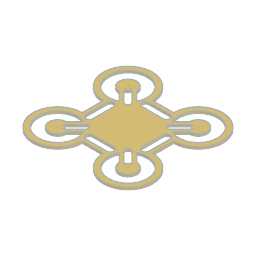
drone (Autodesk Fusion 360 archive; units mm, degrees)
design "body"
part number: 2026-07-30-17-30-24-029
Autodesk Fusion 360 part; units mm, degrees
sketch "Sketch1" plane through (0, 0, 0) normal (0, 1, 0) x (1, 0, 0)
  circle A0 centre (0, 0) radius 35
  circle A1 centre (100, 0.0136) radius 35
  circle A2 centre (0, 100) radius 35
  circle A3 centre (100.1584, 100.0135) radius 35
  line L0 (0, 0) -> (100.1584, 0)
  line L1 (100.1584, 0) -> (100.1584, 100.0135)
  line L2 (100.1584, 100.0135) -> (0, 100.0135)
  line L3 (0, 100.0135) -> (0, 0)
  circle A4 centre (0, 0) radius 27.5
  circle A5 centre (100, 0.0136) radius 27.5
  circle A6 centre (100.1584, 100.0135) radius 27.5
  circle A7 centre (0, 100) radius 27.5
  circle A8 centre (100.1584, 100.0135) radius 12.5
  circle A9 centre (0, 100) radius 12.5
  circle A10 centre (100, 0.0136) radius 12.5
  circle A11 centre (0, 0) radius 12.5
  line L4 (0, 12.5) -> (21.9203, 34.4203)
  line L5 (21.9203, 34.4203) -> (34.4203, 21.9203)
  line L6 (34.4203, 21.9203) -> (12.5, 0)
  line L7 (0, 12.5) -> (12.5, 0)
  line L8 (87.5, 0) -> (65.707, 22.0469)
  line L9 (65.707, 22.0469) -> (78.3654, 34.5595)
  line L10 (78.3654, 34.5595) -> (100.1584, 12.5126)
  line L11 (87.5, 0) -> (100.1584, 12.5126)
  line L12 (0, 87.5) -> (12.5, 100.0135)
  line L13 (0, 87.5) -> (21.9321, 65.5915)
  line L14 (21.9321, 65.5915) -> (34.4321, 78.105)
  line L15 (34.4321, 78.105) -> (12.5, 100.0135)
  line L16 (87.6584, 100.0135) -> (100.1584, 87.5135)
  line L17 (100.1584, 87.5135) -> (78.2381, 65.5932)
  line L18 (87.6584, 100.0135) -> (65.7381, 78.0932)
  line L19 (65.7381, 78.0932) -> (78.2381, 65.5932)
  dimension "d1" = 70
  dimension "d2" = 70
  dimension "d3" = 70
  dimension "d4" = 70
  dimension "d5" = 100
  dimension "d6" = 100
  dimension "d7" = 100
  dimension "d8" = 55
  dimension "d9" = 55
  dimension "d10" = 55
  dimension "d11" = 55
  dimension "d12" = 25
  dimension "d13" = 25
  dimension "d14" = 25
  dimension "d15" = 25
  dimension "d16" = 31
  dimension "d17" = 31
  dimension "d18" = 31
  dimension "d19" = 31
  constraint coincident A0.centre L0.start
  constraint horizontal L0
  constraint vertical L1
  constraint horizontal L2
  constraint vertical L3
  constraint coincident A3.centre L1.end
  constraint concentric A0 A4
  constraint concentric A1 A5
  constraint concentric A3 A6
  constraint concentric A2 A7
  constraint concentric A3 A8
  constraint concentric A2 A9
  constraint concentric A5 A10
  constraint coincident L3 L4.start
  constraint coincident A11 L4.start
  constraint coincident A11 L6.end
  constraint coincident L0 L6.end
  constraint perpendicular L5 L6
  constraint perpendicular L4 L5
  constraint parallel L5 L7
  constraint coincident A10 L8.start
  constraint coincident L0 L8.start
  constraint coincident A10 L10.end
  constraint coincident L1 L10.end
  constraint parallel L9 L11
  constraint perpendicular L8 L11
  constraint perpendicular L9 L10
  constraint coincident A9 L12.start
  constraint coincident L3 L12.start
  constraint coincident A9 L12.end
  constraint coincident L2 L12.end
  constraint perpendicular L12 L13
  constraint perpendicular L13 L14
  constraint perpendicular L14 L15
  constraint coincident A8 L16.start
  constraint coincident L2 L16.start
  constraint coincident L1 L16.end
  constraint coincident A8 L16.end
  constraint coincident L16 L18.start
  constraint perpendicular L18 L19
  constraint perpendicular L17 L19
  constraint parallel L16 L19
  measures "d1" diameter of A0
  measures "d2" diameter of A1
  measures "d3" diameter of A2
  measures "d4" diameter of A3
  measures "d5" distance of A1.centre A3.centre
  measures "d6" distance of A0.centre A1.centre
  measures "d7" distance of A0.centre A2.centre
  measures "d8" diameter of A4
  measures "d9" diameter of A5
  measures "d10" diameter of A6
  measures "d11" diameter of A7
  measures "d12" diameter of A8
  measures "d13" diameter of A9
  measures "d14" diameter of A10
  measures "d15" diameter of A11
  measures "d16" distance of L5.end L6.end
  measures "d17" distance of L8.start L8.end
  measures "d18" distance of L12.end L14.end
  measures "d19" distance of L16.end L17.end
extrude "Extrude1" add sketch "Sketch1" along normal blind 3 contours A0 L0 A4 L6 | A0 L0 L3 A4 | A0 A1 A2 A3 L0 L1 L2 L3 L4 L5 L6 L8 L9 L10 L13 L14 L15 L17 L18 L19 | A0 A4 L4 L6 | A0 L4 L5 L6 | A0 L3 A4 L4 | A1 L0 L1 A5 | A1 L0 A5 L8 | A4 A11 L4 L6 | A2 L3 A7 L13 | A2 L2 L3 A7 | L0 L3 A11 | A11 L7 | L0 L3 L7 | A1 L8 L9 L10 | A1 A5 L8 L10 | A2 L2 A7 L15 | A2 A7 L13 L15 | A2 L13 L14 L15 | A1 L1 A5 L10 | A5 A10 L8 L10 | L0 L1 L11 | L0 L1 A10 | A10 L11 | A3 L2 A6 L18 | A3 L1 L2 A6 | A7 A9 L13 L15 | L2 L3 A9 | A9 L12 | L2 L3 L12 | A3 L1 A6 L17 | A3 A6 L17 L18 | A3 L17 L18 L19 | A6 A8 L17 L18 | L1 L2 A8 | A8 L16 | L1 L2 L16
move_face "MoveFace1" by (0, 0, 90) 1 faces at (58.5153, 0, -62.6556)
move_body "Move1" bodies 1 to x (1, 0, 0) y (0, 0, -1) z (0, 1, 0) at (0, 49.9918, 80.0082)
sketch "Sketch2" plane through (0, 0, 80.0082) normal (0, 0, 1) x (-1, 0, 0)
  line L0 (-100.1584, 37.5217) -> (-87.9948, 25.3581)
  arc A0 (-75.4948, 37.8581) -> (-87.9948, 25.3581) centre (-100.1584, 50.0217) ccw
  line L1 (-75.4948, 37.8581) -> (-87.6584, 50.0217)
  arc A1 (-87.6584, 50.0217) -> (-100.1584, 37.5217) centre (-100.1584, 50.0217) ccw
  line L2 (0, -37.4918) -> (-12.1636, -25.3281)
  arc A2 (-24.6636, -37.8281) -> (-12.1636, -25.3281) centre (0, -49.9918) ccw
  line L3 (-24.6636, -37.8281) -> (-12.5, -49.9918)
  arc A3 (-12.5, -49.9918) -> (0, -37.4918) centre (0, -49.9918) ccw
  line L4 (-12.5, 50.0217) -> (-24.6724, 37.8624)
  arc A4 (-12.1725, 25.3489) -> (-24.6724, 37.8624) centre (0, 50.0082) ccw
  line L5 (-12.1725, 25.3489) -> (0, 37.5082)
  arc A5 (0, 37.5082) -> (-12.5, 50.0217) centre (0, 50.0082) ccw
  line L6 (-87.5, -49.9918) -> (-75.3786, -37.7292)
  arc A6 (-88.037, -25.2165) -> (-75.3786, -37.7292) centre (-100, -49.9781) ccw
  line L7 (-88.037, -25.2165) -> (-100.1584, -37.4791)
  arc A7 (-100.1584, -37.4791) -> (-87.5, -49.9918) centre (-100, -49.9781) ccw
  arc A8 (0, 15.0082) -> (-35, 50.0217) centre (0, 50.0082) ccw
  line L8 (-35, 50.0217) -> (-65.1584, 50.0217)
  arc A9 (-65.1584, 50.0217) -> (-100.1584, 15.0217) centre (-100.1584, 50.0217) ccw
  line L9 (-100.1584, 15.0217) -> (-100.1584, -14.9785)
  arc A10 (-100.1584, -14.9785) -> (-65, -49.9918) centre (-100, -49.9781) ccw
  line L10 (-65, -49.9918) -> (-35, -49.9918)
  arc A11 (-35, -49.9918) -> (0, -14.9918) centre (0, -49.9918) ccw
  line L11 (0, -14.9918) -> (0, 15.0082)
  line L12 (-35, -35) -> (-65, -35)
  arc A12 (-65, -35) -> (-65, -45) centre (-65, -40) ccw
  line L13 (-65, -45) -> (-35, -45)
  arc A13 (-35, -45) -> (-35, -35) centre (-35, -40) ccw
  line L14 (-35, -40) -> (-65, -40) construction
  line L15 (-35, 45) -> (-65, 45)
  arc A14 (-65, 45) -> (-65, 35) centre (-65, 40) ccw
  line L16 (-65, 35) -> (-35, 35)
  arc A15 (-35, 35) -> (-35, 45) centre (-35, 40) ccw
  line L17 (-35, 40) -> (-65, 40) construction
  line L18 (-15, 15) -> (-15, -15)
  arc A16 (-15, -15) -> (-5, -15) centre (-10, -15) ccw
  line L19 (-5, -15) -> (-5, 15)
  arc A17 (-5, 15) -> (-15, 15) centre (-10, 15) ccw
  line L20 (-10, 15) -> (-10, -15) construction
  line L21 (-95, 15) -> (-95, -15)
  arc A18 (-95, -15) -> (-85, -15) centre (-90, -15) ccw
  line L22 (-85, -15) -> (-85, 15)
  arc A19 (-85, 15) -> (-95, 15) centre (-90, 15) ccw
  line L23 (-90, 15) -> (-90, -15) construction
  dimension "d22" = 10
  dimension "d23" = 10
  constraint tangent L12 A12
  constraint tangent A12 L13
  constraint parallel L12 L13
  constraint tangent L13 A13
  constraint tangent L12 A13
  constraint horizontal L14
  constraint tangent L15 A14
  constraint tangent A14 L16
  constraint parallel L15 L16
  constraint tangent L16 A15
  constraint tangent L15 A15
  constraint parallel L12 L17
  constraint tangent L18 A16
  constraint tangent A16 L19
  constraint parallel L18 L19
  constraint tangent L19 A17
  constraint tangent L18 A17
  constraint vertical L20
  constraint tangent L21 A18
  constraint tangent A18 L22
  constraint parallel L21 L22
  constraint tangent L22 A19
  constraint tangent L21 A19
  constraint parallel L9 L23
  measures "d22" diameter of A14
  measures "d23" diameter of A18
extrude "Extrude2" cut sketch "Sketch2" against normal blind 40 contours L12 A12 L13 A13 | L15 A14 L16 A15 | L18 A16 L19 A17 | L21 A18 L22 A19
sketch "Sketch3" plane through (0, 0, 80.0082) normal (0, 0, 1) x (-1, 0, 0)
  arc A0 (0, 15.0082) -> (-35, 50.0217) centre (0, 50.0082) ccw
  line L0 (-35, 50.0217) -> (-65.1584, 50.0217)
  arc A1 (-65.1584, 50.0217) -> (-100.1584, 15.0217) centre (-100.1584, 50.0217) ccw
  line L1 (-100.1584, 15.0217) -> (-100.1584, -14.9785)
  arc A2 (-100.1584, -14.9785) -> (-65, -49.9918) centre (-100, -49.9781) ccw
  line L2 (-65, -49.9918) -> (-35, -49.9918)
  arc A3 (-35, -49.9918) -> (0, -14.9918) centre (0, -49.9918) ccw
  line L3 (0, -14.9918) -> (0, 15.0082)
  line L4 (-87.5, -49.9918) -> (-75.3786, -37.7292)
  arc A4 (-88.037, -25.2165) -> (-75.3786, -37.7292) centre (-100, -49.9781) ccw
  line L5 (-88.037, -25.2165) -> (-100.1584, -37.4791)
  arc A5 (-100.1584, -37.4791) -> (-87.5, -49.9918) centre (-100, -49.9781) ccw
  line L6 (-12.5, 50.0217) -> (-24.6724, 37.8624)
  arc A6 (-12.1725, 25.3489) -> (-24.6724, 37.8624) centre (0, 50.0082) ccw
  line L7 (-12.1725, 25.3489) -> (0, 37.5082)
  arc A7 (0, 37.5082) -> (-12.5, 50.0217) centre (0, 50.0082) ccw
  line L8 (0, -37.4918) -> (-12.1636, -25.3281)
  arc A8 (-24.6636, -37.8281) -> (-12.1636, -25.3281) centre (0, -49.9918) ccw
  line L9 (-24.6636, -37.8281) -> (-12.5, -49.9918)
  arc A9 (-12.5, -49.9918) -> (0, -37.4918) centre (0, -49.9918) ccw
  line L10 (-100.1584, 37.5217) -> (-87.9948, 25.3581)
  arc A10 (-75.4948, 37.8581) -> (-87.9948, 25.3581) centre (-100.1584, 50.0217) ccw
  line L11 (-75.4948, 37.8581) -> (-87.6584, 50.0217)
  arc A11 (-87.6584, 50.0217) -> (-100.1584, 37.5217) centre (-100.1584, 50.0217) ccw
  line L12 (-65, 45) -> (-35, 45)
  arc A12 (-35, 35) -> (-35, 45) centre (-35, 40) ccw
  line L13 (-35, 35) -> (-65, 35)
  arc A13 (-65, 45) -> (-65, 35) centre (-65, 40) ccw
  line L14 (-95, -15) -> (-95, 15)
  arc A14 (-85, 15) -> (-95, 15) centre (-90, 15) ccw
  line L15 (-85, 15) -> (-85, -15)
  arc A15 (-95, -15) -> (-85, -15) centre (-90, -15) ccw
  line L16 (-15, -15) -> (-15, 15)
  arc A16 (-5, 15) -> (-15, 15) centre (-10, 15) ccw
  line L17 (-5, 15) -> (-5, -15)
  arc A17 (-15, -15) -> (-5, -15) centre (-10, -15) ccw
  line L18 (-65, -35) -> (-35, -35)
  arc A18 (-35, -45) -> (-35, -35) centre (-35, -40) ccw
  line L19 (-35, -45) -> (-65, -45)
  arc A19 (-65, -35) -> (-65, -45) centre (-65, -40) ccw
  line L20 (-7.8284, 47.8284) -> (-22.8284, 32.8284)
  arc A20 (-22.8284, 32.8284) -> (-17.1716, 27.1716) centre (-20, 30) ccw
  line L21 (-17.1716, 27.1716) -> (-2.1716, 42.1716)
  arc A21 (-2.1716, 42.1716) -> (-7.8284, 47.8284) centre (-5, 45) ccw
  line L22 (-5, 45) -> (-20, 30) construction
  line L23 (-97.8284, 42.1716) -> (-82.8284, 27.1716)
  arc A22 (-82.8284, 27.1716) -> (-77.1716, 32.8284) centre (-80, 30) ccw
  line L24 (-77.1716, 32.8284) -> (-92.1716, 47.8284)
  arc A23 (-92.1716, 47.8284) -> (-97.8284, 42.1716) centre (-95, 45) ccw
  line L25 (-95, 45) -> (-80, 30) construction
  line L26 (-92.1552, -47.812) -> (-77.2438, -32.7268)
  arc A24 (-77.2438, -32.7268) -> (-82.9333, -27.1028) centre (-80.0885, -29.9148) ccw
  line L27 (-82.9333, -27.1028) -> (-97.8448, -42.188)
  arc A25 (-97.8448, -42.188) -> (-92.1552, -47.812) centre (-95, -45) ccw
  line L28 (-95, -45) -> (-80.0885, -29.9148) construction
  line L29 (-2.1716, -42.1716) -> (-17.1716, -27.1716)
  arc A26 (-17.1716, -27.1716) -> (-22.8284, -32.8284) centre (-20, -30) ccw
  line L30 (-22.8284, -32.8284) -> (-7.8284, -47.8284)
  arc A27 (-7.8284, -47.8284) -> (-2.1716, -42.1716) centre (-5, -45) ccw
  line L31 (-5, -45) -> (-20, -30) construction
  line L32 (-5, -45) -> (-2.1716, -42.1716)
  line L33 (-5, -45) -> (-7.8284, -47.8284)
  line L34 (-95, -45) -> (-92.1552, -47.812)
  line L35 (-95, -45) -> (-97.8448, -42.188)
  line L36 (-95, 45) -> (-92.1716, 47.8284)
  line L37 (-95, 45) -> (-97.8284, 42.1716)
  line L38 (-5, 45) -> (-7.8284, 47.8284)
  line L39 (-5, 45) -> (-2.1716, 42.1716)
  dimension "d26" = 8
  dimension "d27" = 8
  dimension "d28" = 8
  dimension "d29" = 8
  constraint tangent L20 A20
  constraint tangent A20 L21
  constraint parallel L20 L21
  constraint tangent L21 A21
  constraint tangent L20 A21
  constraint tangent L23 A22
  constraint tangent A22 L24
  constraint parallel L23 L24
  constraint tangent L24 A23
  constraint tangent L23 A23
  constraint tangent L26 A24
  constraint tangent A24 L27
  constraint parallel L26 L27
  constraint tangent L27 A25
  constraint tangent L26 A25
  constraint parallel L4 L28
  constraint tangent L29 A26
  constraint tangent A26 L30
  constraint parallel L29 L30
  constraint tangent L30 A27
  constraint tangent L29 A27
  constraint coincident A27.centre L31.start
  constraint coincident A25.centre L28.start
  constraint coincident A23.centre L25.start
  constraint coincident A21.centre L22.start
  measures "d26" diameter of A20
  measures "d27" diameter of A22
  measures "d28" diameter of A24
  measures "d29" diameter of A26
extrude "Extrude3" cut sketch "Sketch3" against normal blind 3 contours L20 A20 L21 L38 L39 | L23 A22 L24 L36 L37 | L26 A24 L27 L34 L35 | L29 A26 L30 L32 L33
sketch "Sketch4" plane through (0, 0, 80.0082) normal (0, 0, 1) x (-1, 0, 0)
  line L0 (-65, -35) -> (-35, -35)
  arc A0 (-35, -45) -> (-35, -35) centre (-35, -40) ccw
  line L1 (-35, -45) -> (-65, -45)
  arc A1 (-65, -35) -> (-65, -45) centre (-65, -40) ccw
  line L2 (-15, -15) -> (-15, 15)
  arc A2 (-5, 15) -> (-15, 15) centre (-10, 15) ccw
  line L3 (-5, 15) -> (-5, -15)
  arc A3 (-15, -15) -> (-5, -15) centre (-10, -15) ccw
  line L4 (-95, -15) -> (-95, 15)
  arc A4 (-85, 15) -> (-95, 15) centre (-90, 15) ccw
  line L5 (-85, 15) -> (-85, -15)
  arc A5 (-95, -15) -> (-85, -15) centre (-90, -15) ccw
  line L6 (-65, 45) -> (-35, 45)
  arc A6 (-35, 35) -> (-35, 45) centre (-35, 40) ccw
  line L7 (-35, 35) -> (-65, 35)
  arc A7 (-65, 45) -> (-65, 35) centre (-65, 40) ccw
  line L8 (-100.1584, 37.5217) -> (-87.9948, 25.3581)
  arc A8 (-75.4948, 37.8581) -> (-87.9948, 25.3581) centre (-100.1584, 50.0217) ccw
  line L9 (-75.4948, 37.8581) -> (-87.6584, 50.0217)
  arc A9 (-87.6584, 50.0217) -> (-100.1584, 37.5217) centre (-100.1584, 50.0217) ccw
  line L10 (0, -37.4918) -> (-12.1636, -25.3281)
  arc A10 (-24.6636, -37.8281) -> (-12.1636, -25.3281) centre (0, -49.9918) ccw
  line L11 (-24.6636, -37.8281) -> (-12.5, -49.9918)
  arc A11 (-12.5, -49.9918) -> (0, -37.4918) centre (0, -49.9918) ccw
  line L12 (-12.5, 50.0217) -> (-24.6724, 37.8624)
  arc A12 (-12.1725, 25.3489) -> (-24.6724, 37.8624) centre (0, 50.0082) ccw
  line L13 (-12.1725, 25.3489) -> (0, 37.5082)
  arc A13 (0, 37.5082) -> (-12.5, 50.0217) centre (0, 50.0082) ccw
  line L14 (-87.5, -49.9918) -> (-75.3786, -37.7292)
  arc A14 (-88.037, -25.2165) -> (-75.3786, -37.7292) centre (-100, -49.9781) ccw
  line L15 (-88.037, -25.2165) -> (-100.1584, -37.4791)
  arc A15 (-100.1584, -37.4791) -> (-87.5, -49.9918) centre (-100, -49.9781) ccw
  arc A16 (0, 15.0082) -> (-35, 50.0217) centre (0, 50.0082) ccw
  line L16 (-35, 50.0217) -> (-65.1584, 50.0217)
  arc A17 (-65.1584, 50.0217) -> (-100.1584, 15.0217) centre (-100.1584, 50.0217) ccw
  line L17 (-100.1584, 15.0217) -> (-100.1584, -14.9785)
  arc A18 (-100.1584, -14.9785) -> (-65, -49.9918) centre (-100, -49.9781) ccw
  line L18 (-65, -49.9918) -> (-35, -49.9918)
  arc A19 (-35, -49.9918) -> (0, -14.9918) centre (0, -49.9918) ccw
  line L19 (0, -14.9918) -> (0, 15.0082)
  line L20 (-82.8284, 27.1716) -> (-97.8284, 42.1716)
  line L21 (-97.8284, 42.1716) -> (-92.1716, 47.8284)
  line L22 (-92.1716, 47.8284) -> (-77.1716, 32.8284)
  arc A20 (-82.8284, 27.1716) -> (-77.1716, 32.8284) centre (-80, 30) ccw
  arc A21 (-77.2438, -32.7268) -> (-82.9333, -27.1028) centre (-80.0885, -29.9148) ccw
  line L23 (-77.2438, -32.7268) -> (-92.1552, -47.812)
  line L24 (-92.1552, -47.812) -> (-97.8448, -42.188)
  line L25 (-97.8448, -42.188) -> (-82.9333, -27.1028)
  arc A22 (-22.8284, 32.8284) -> (-17.1716, 27.1716) centre (-20, 30) ccw
  line L26 (-22.8284, 32.8284) -> (-7.8284, 47.8284)
  line L27 (-7.8284, 47.8284) -> (-2.1716, 42.1716)
  line L28 (-2.1716, 42.1716) -> (-17.1716, 27.1716)
  arc A23 (-17.1716, -27.1716) -> (-22.8284, -32.8284) centre (-20, -30) ccw
  line L29 (-17.1716, -27.1716) -> (-2.1716, -42.1716)
  line L30 (-2.1716, -42.1716) -> (-7.8284, -47.8284)
  line L31 (-7.8284, -47.8284) -> (-22.8284, -32.8284)
sketch "Sketch5" plane through (0, 0, 80.0082) normal (0, 0, 1) x (1, 0, 0)
  line L0 (0, 14.9918) -> (0, -15.0082)
  arc A0 (0, -15.0082) -> (35, -50.0217) centre (0, -50.0082) ccw
  arc A1 (12.1725, -25.3489) -> (24.6724, -37.8624) centre (0, -50.0082) ccw
  arc A2 (0, -37.5082) -> (12.5, -50.0217) centre (0, -50.0082) ccw
  line L1 (12.1725, -25.3489) -> (0, -37.5082)
  circle A3 centre (0, -50.0082) radius 0.7
  circle A4 centre (1.7574, -44.0082) radius 0.7
  line L2 (1.7574, -44.0082) -> (7, -44.0082) construction
  circle A5 centre (6, -48.2509) radius 0.7
  circle A6 centre (100, 50) radius 0.7
  circle A7 centre (98.4213, 44.2114) radius 0.7
  line L3 (98.4213, 44.2114) -> (104.4213, 44.2114) construction
  circle A8 centre (94.201, 48.46) radius 0.7
  circle A9 centre (100, -50.4942) radius 0.7
  circle A10 centre (94, -49) radius 0.7
  line L4 (94, -49) -> (100, -49) construction
  circle A11 centre (98.2426, -44.7574) radius 0.7
  circle A12 centre (0, 50.4942) radius 0.7
  circle A13 centre (6, 49) radius 0.7
  circle A14 centre (1.7574, 44.7574) radius 0.7
  dimension "d32" = 30
  dimension "d33" = 35
  dimension "d34" = 27.5
  dimension "d35" = 12.5
  dimension "d36" = 17.2052
  dimension "d37" = 1.4
  dimension "d38" = 1.4
  dimension "d39" = 6
  dimension "d40" = 6
  dimension "d42" = 1.4
  dimension "d43" = 6
  dimension "d44" = 1.4
  dimension "d45" = 1.4
  dimension "d47" = 6
  dimension "d50" = 1.4
  dimension "d51" = 5.9884
  dimension "d52" = 6
  dimension "d53" = 1.4
  dimension "d54" = 1.4
  dimension "d55" = 6
  dimension "d58" = 1.4
  dimension "d59" = 6
  dimension "d60" = 6
  dimension "d61" = 1.4
  dimension "d62" = 1.4
  dimension "d63" = 6
  dimension "d64" = 6
  dimension "d65" = 1.4
  dimension "d66" = 6
  constraint concentric A0 A3
  constraint horizontal L2
  constraint coincident A4.centre L2.start
  constraint horizontal L3
  constraint coincident A7.centre L3.start
  constraint horizontal L4
  constraint coincident A10.centre L4.start
  measures "d32" distance of L0.start L0.end
  measures "d33" radius of A0
  measures "d34" radius of A1
  measures "d35" radius of A2
  measures "d36" distance of A1.start A2.start
  measures "d37" diameter of A3
  measures "d38" diameter of A4
  measures "d39" vertical distance of A0.centre A4.centre
  measures "d40" distance of A4.centre A5.centre
  measures "d42" diameter of A5
  measures "d43" horizontal distance of A0.centre A5.centre
  measures "d44" diameter of A6
  measures "d45" diameter of A7
  measures "d47" distance of A6.centre A7.centre
  measures "d50" diameter of A8
  measures "d51" distance of A7.centre A8.centre
  measures "d52" distance of A6.centre A8.centre
  measures "d53" diameter of A9
  measures "d54" diameter of A10
  measures "d55" horizontal distance of A9.centre A10.centre
  measures "d58" diameter of A11
  measures "d59" distance of A10.centre A11.centre
  measures "d60" distance of A9.centre A11.centre
  measures "d61" diameter of A12
  measures "d62" diameter of A13
  measures "d63" horizontal distance of A12.centre A13.centre
  measures "d64" distance of A13.centre A14.centre
  measures "d65" diameter of A14
  measures "d66" distance of A12.centre A14.centre
extrude "Extrude4" cut sketch "Sketch5" against normal blind 5
sketch "Sketch6" plane through (0, 0, 80.0082) normal (0, 0, 1) x (-1, 0, 0)
sketch "Sketch7" plane through (0, 0, 80.0082) normal (0, 0, 1) x (-1, 0, 0)
